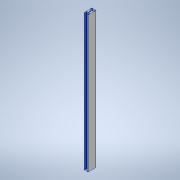
# Autodesk Inventor part: I330
Saved by Autodesk Inventor 2021.1 (Build 251245010, 245A)
## iProperties
Created: 2019-08-30
Part Number: I330
Material: アルミニウム 6061
Document SubType Name: Modeling
Designer: gisen
Density: 2.7 g/cm^3
Appearance: アルミニウム - フラット
Author: gisen
Autodesk Inventor part; units mm, degrees
ref_plane "YZ Plane" through (0, 0, 0) normal (1, 0, 0) x (0, 1, 0)
ref_plane "XZ Plane" through (0, 0, 0) normal (0, 1, 0) x (-1, 0, 0)
ref_plane "XY Plane" through (0, 0, 0) normal (0, 0, 1) x (1, 0, 0)
sketch "BaseI" plane through (0, 0, 0) normal (0, 0, 1) x (1, 0, 0)
  line L0 (-4.5, -10) -> (-2.65, -10)
  line L1 (5, -9.5) -> (5, 9.5)
  line L2 (4.5, 10) -> (2.65, 10)
  line L3 (-5, 9.5) -> (-5, -9.5)
  line L4 (-5, -10) -> (5, 10) construction
  line L5 (5, -10) -> (-5, 10) construction
  line L6 (3.85, 8.5) -> (2.65, 8.5)
  line L7 (-4.15, 8.2) -> (-4.15, 5.1)
  line L8 (-3.85, 4.8) -> (-2.65, 4.8)
  line L9 (4.15, 5.1) -> (4.15, 8.2)
  line L10 (4.15, 8.5) -> (-4.15, 4.8) construction
  line L11 (-4.15, 8.5) -> (4.15, 4.8) construction
  line L12 (-1.55, 3) -> (1.55, 3)
  line L13 (2.15, 3.6) -> (2.15, 4.3)
  line L14 (-2.15, 9.5) -> (-2.15, 9)
  line L15 (-2.15, 3) -> (2.15, 10) construction
  line L16 (2.15, 3) -> (-2.15, 10) construction
  line L17 (3.85, -8.5) -> (2.65, -8.5)
  line L18 (-4.15, -8.2) -> (-4.15, -5.1)
  line L19 (-3.85, -4.8) -> (-2.65, -4.8)
  line L20 (4.15, -5.1) -> (4.15, -8.2)
  line L21 (4.15, -8.5) -> (-4.15, -4.8) construction
  line L22 (-4.15, -8.5) -> (4.15, -4.8) construction
  line L23 (1.55, -3) -> (-1.55, -3)
  line L24 (-2.15, -3.6) -> (-2.15, -4.3)
  line L25 (2.15, -9.5) -> (2.15, -9)
  line L26 (2.15, -3) -> (-2.15, -10) construction
  line L27 (-2.15, -3) -> (2.15, -10) construction
  arc A0 (-4.5, 10) -> (-5, 9.5) centre (-4.5, 9.5) ccw
  arc A1 (5, 9.5) -> (4.5, 10) centre (4.5, 9.5) ccw
  arc A2 (4.5, -10) -> (5, -9.5) centre (4.5, -9.5) ccw
  arc A3 (-5, -9.5) -> (-4.5, -10) centre (-4.5, -9.5) ccw
  line L28 (-2.65, 10) -> (-4.5, 10)
  line L29 (2.65, -10) -> (4.5, -10)
  arc A4 (-3.85, 8.5) -> (-4.15, 8.2) centre (-3.85, 8.2) ccw
  arc A5 (-4.15, 5.1) -> (-3.85, 4.8) centre (-3.85, 5.1) ccw
  arc A6 (4.15, 8.2) -> (3.85, 8.5) centre (3.85, 8.2) ccw
  arc A7 (3.85, 4.8) -> (4.15, 5.1) centre (3.85, 5.1) ccw
  arc A8 (-3.85, -4.8) -> (-4.15, -5.1) centre (-3.85, -5.1) ccw
  arc A9 (-4.15, -8.2) -> (-3.85, -8.5) centre (-3.85, -8.2) ccw
  arc A10 (4.15, -5.1) -> (3.85, -4.8) centre (3.85, -5.1) ccw
  arc A11 (3.85, -8.5) -> (4.15, -8.2) centre (3.85, -8.2) ccw
  arc A12 (-2.15, 3.6) -> (-1.55, 3) centre (-1.55, 3.6) ccw
  arc A13 (1.55, 3) -> (2.15, 3.6) centre (1.55, 3.6) ccw
  arc A14 (-1.55, -3) -> (-2.15, -3.6) centre (-1.55, -3.6) ccw
  arc A15 (2.15, -3.6) -> (1.55, -3) centre (1.55, -3.6) ccw
  arc A16 (-2.15, 9.5) -> (-2.65, 10) centre (-2.65, 9.5) ccw
  arc A17 (2.65, 10) -> (2.15, 9.5) centre (2.65, 9.5) ccw
  line L30 (-2.65, 8.5) -> (-3.85, 8.5)
  line L31 (2.65, 4.8) -> (3.85, 4.8)
  line L32 (2.15, 9) -> (2.15, 9.5)
  line L33 (-2.15, 4.3) -> (-2.15, 3.6)
  line L34 (2.15, -4.3) -> (2.15, -3.6)
  line L35 (-2.15, -9) -> (-2.15, -9.5)
  line L36 (2.65, -4.8) -> (3.85, -4.8)
  line L37 (-2.65, -8.5) -> (-3.85, -8.5)
  arc A18 (-2.15, 4.3) -> (-2.65, 4.8) centre (-2.65, 4.3) ccw
  arc A19 (2.65, 4.8) -> (2.15, 4.3) centre (2.65, 4.3) ccw
  arc A20 (2.15, 9) -> (2.65, 8.5) centre (2.65, 9) ccw
  arc A21 (-2.65, 8.5) -> (-2.15, 9) centre (-2.65, 9) ccw
  arc A22 (-2.65, -4.8) -> (-2.15, -4.3) centre (-2.65, -4.3) ccw
  arc A23 (2.15, -4.3) -> (2.65, -4.8) centre (2.65, -4.3) ccw
  arc A24 (2.65, -8.5) -> (2.15, -9) centre (2.65, -9) ccw
  arc A25 (-2.15, -9) -> (-2.65, -8.5) centre (-2.65, -9) ccw
  arc A26 (-2.65, -10) -> (-2.15, -9.5) centre (-2.65, -9.5) ccw
  arc A27 (2.15, -9.5) -> (2.65, -10) centre (2.65, -9.5) ccw
  circle A28 centre (0, 0) radius 1.65
  point P0 (0, 6.65)
  point P1 (0, 6.5)
  point P2 (0, -6.65)
  point P3 (0, -6.5)
  point P4 (0, 6.5)
  point P5 (0, 10)
  point P6 (0, -6.5)
  point P7 (0, -10)
  point P8 (0, 6.65)
  point P9 (0, 10)
  point P10 (0, 6.65)
  point P11 (0, -6.65)
  point P12 (0, -10)
  point P13 (0, -6.5)
  point P14 (0, -6.65)
  point P15 (0, 6.5)
  dimension "d0" = 10
  dimension "d1" = 20
  dimension "d2" = 7
  dimension "d3" = 4.3
  dimension "d4" = 7
  dimension "d5" = 4.3
  dimension "d6" = 8.3
  dimension "d7" = 8.3
  dimension "d8" = 3.7
  dimension "d9" = 3.7
  dimension "d10" = 1.5
  dimension "d11" = 1.5
  dimension "d12" = 0.5
  dimension "d13" = 0.3
  dimension "d14" = 0.6
  dimension "d15" = 0.5
  dimension "d16" = 0.5
  dimension "d17" = 3.3
  constraints: 76 end point, 74 tangent, 56 point on circle, 40 point on line, 29 centre point, 23 equal radius, 23 parallel, 21 midpoint, 10 perpendicular, 8 horizontal, 8 vertical alignment
  measures "d0" distance of L5.end L4.end
  measures "d1" distance of L4.end L5.start
  measures "d2" distance of L16.start L15.end
  measures "d3" distance of L15.start L16.start
  measures "d4" distance of L27.end L26.start
  measures "d5" distance of L26.start L27.start
  measures "d6" distance of L10.end L11.end
  measures "d7" distance of L21.end L22.end
  measures "d8" distance of L11.end L10.start
  measures "d9" distance of L22.end L21.start
  measures "d10" distance between parallel lines of L6 L2
  measures "d11" distance between parallel lines of L0 L17
  measures "d12" radius of A0
  measures "d13" radius of A4
  measures "d14" radius of A12
  measures "d15" radius of A16
  measures "d16" radius of A18
  measures "d17" diameter of A28
extrude "押し出し1" add sketch "BaseI" along normal blind 330
